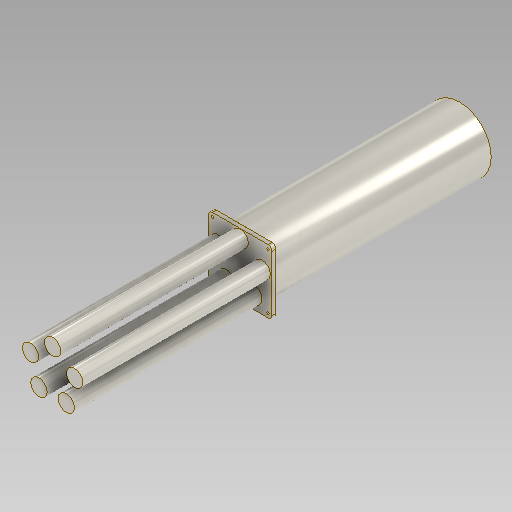
# Autodesk Inventor part: atornillador
Saved by Autodesk Inventor 2021 (Build 250183000, 183)
## iProperties
Created: 2022-02-01
Part Number: atornillador
Material: Acerito
Document SubType Name: Modeling
Designer: Osmar Ediber Toloza Bernal
Density: 8 g/cm^3
Appearance: Titanio
Mass: 114460 g
Surface Area: 6362.52 cm^2
Volume: 14307.5 cm^3
Author: Osmar Ediber Toloza Bernal
Autodesk Inventor part; units mm, degrees
ref_plane "YZ Plane" through (0, 0, 0) normal (1, 0, 0) x (0, 1, 0)
ref_plane "XZ Plane" through (0, 0, 0) normal (0, 1, 0) x (-1, 0, 0)
ref_plane "XY Plane" through (0, 0, 0) normal (0, 0, 1) x (1, 0, 0)
sketch "Boceto1" plane through (0, 0, 0) normal (0, 0, 1) x (1, 0, 0)
  circle A0 centre (0, 0) radius 80
  dimension "d0" = 160
  constraints: 1 centre point, 1 coincident
  measures "d0" diameter of A0
extrude "Extrusión1" add sketch "Boceto1" against normal blind 542
sketch "Boceto2" plane through (0, 0, 0) normal (0, 0, 1) x (1, 0, 0)
  line L0 (-70, 80) -> (70, 80)
  line L1 (80, 70) -> (80, -70)
  line L2 (70, -80) -> (-70, -80)
  line L3 (-80, -70) -> (-80, 70)
  circle A0 centre (0, 0) radius 80 construction
  circle A1 centre (-70, 70) radius 3
  arc A2 (-70, 80) -> (-80, 70) centre (-70, 70) ccw
  arc A3 (80, 70) -> (70, 80) centre (70, 70) ccw
  arc A4 (70, -80) -> (80, -70) centre (70, -70) ccw
  arc A5 (-80, -70) -> (-70, -80) centre (-70, -70) ccw
  circle A6 centre (-70, -70) radius 3
  circle A7 centre (70, -70) radius 3
  circle A8 centre (70, 70) radius 3
  dimension "d4" = 6
  dimension "d5" = 10
  dimension "d6" = 10
  dimension "d7" = 10
  dimension "d10" = 360
  constraints: 12 tangent, 8 centre point, 8 end point, 8 point on circle, 3 equal radius, 2 parallel, 1 horizontal, 1 perpendicular, 9 other
  measures "d4" diameter of A1
  measures "d5" distance from line of L0 A1.centre
  measures "d6" distance from line of L3 A1.centre
  measures "d7" radius of A2
extrude "Extrusión2" add sketch "Boceto2" along normal blind 10
sketch "Boceto3" plane through (0, 0, 10) normal (0, 0, 1) x (1, 0, 0)
  circle A0 centre (0, 0) radius 58.4375 construction
  circle A1 centre (0, 58.4375) radius 20.625
  circle A2 centre (0, 0) radius 58.4375 construction
  circle A3 centre (-55.5774, 18.0582) radius 20.625
  circle A4 centre (0, 0) radius 58.4375 construction
  circle A5 centre (-34.3487, -47.2769) radius 20.625
  circle A6 centre (0, 0) radius 58.4375 construction
  circle A7 centre (34.3487, -47.2769) radius 20.625
  circle A8 centre (0, 0) radius 58.4375 construction
  circle A9 centre (55.5774, 18.0582) radius 20.625
  dimension "d14" = 116.875
  dimension "d15" = 41.25
  dimension "d18" = 360
  constraints: 5 centre point, 1 coincident, 1 vertical alignment, 35 other
  measures "d15" diameter of A1
extrude "Extrusión3" add sketch "Boceto3" along normal blind 472.3
equation "\"d1\" = 2 * ancho_llanta"
equation "\"d6\" = d5"
equation "\"ancho_llanta\" = 271"
